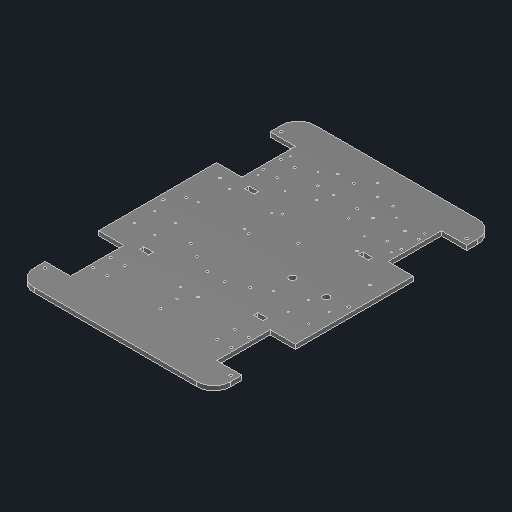
# Autodesk Inventor part: 부품7
Saved by Autodesk Inventor 2026.1 (Build 301233020, 233B)
## iProperties
Created: 2025-11-12
Part Number: 부품7
Material: ABS 플라스틱
Document SubType Name: Modeling
Designer: jaewook
Density: 1.06 g/cm^3
Appearance: 매끄러움 - 흰색
Author: jaewook
Autodesk Inventor part; units mm, degrees
ref_plane "YZ Plane" through (0, 0, 0) normal (1, 0, 0) x (0, 1, 0)
ref_plane "XZ Plane" through (0, 0, 0) normal (0, 1, 0) x (-1, 0, 0)
ref_plane "XY Plane" through (0, 0, 0) normal (0, 0, 1) x (1, 0, 0)
sketch "스케치1" plane through (0, 0, 0) normal (0, 1, 0) x (-1, 0, 0)
  line L0 (145, 250) -> (-145, 250)
  line L1 (-175, 220) -> (-175, -220)
  line L2 (-145, -250) -> (145, -250)
  line L3 (175, -220) -> (175, 220)
  line L4 (175, 250) -> (-175, -250) construction
  line L5 (-175, 250) -> (175, -250) construction
  arc A0 (145, -250) -> (175, -220) centre (145, -220) ccw
  arc A1 (-175, -220) -> (-145, -250) centre (-145, -220) ccw
  arc A2 (-145, 250) -> (-175, 220) centre (-145, 220) ccw
  arc A3 (175, 220) -> (145, 250) centre (145, 220) ccw
  line L6 (0, 0) -> (0, -150)
  line L7 (0, 0) -> (-113, 0)
  line L8 (175, -200) -> (130, -200)
  line L9 (130, -200) -> (130, -105)
  line L10 (130, -105) -> (175, -105)
  line L11 (175, -105) -> (175, -200)
  line L12 (-175, -200) -> (-130, -200)
  line L13 (-130, -200) -> (-130, -105)
  line L14 (-130, -105) -> (-175, -105)
  line L15 (-175, -105) -> (-175, -200)
  line L16 (175, 200) -> (130, 200)
  line L17 (130, 200) -> (130, 105)
  line L18 (130, 105) -> (175, 105)
  line L19 (175, 105) -> (175, 200)
  line L20 (-175, 200) -> (-130, 200)
  line L21 (-130, 105) -> (-175, 105)
  line L22 (-175, 105) -> (-175, 200)
  line L23 (-130, 200) -> (-130, 105)
  point P0 (-175, 200)
  point P1 (-175, 105)
  point P2 (-175, -105)
  point P3 (-175, -200)
  point P4 (175, 105)
  point P5 (175, 200)
  dimension "d0" = 350
  dimension "d1" = 500
  dimension "d2" = 30
  dimension "d4" = 95
  dimension "d5" = 45
  dimension "d6" = 50
  dimension "d9" = 50
  dimension "d10" = 45
  dimension "d11" = 95
  constraints: 48 end point, 12 symmetric about line, 9 point on line, 8 point on circle, 8 tangent, 4 centre point, 4 parallel, 3 equal radius, 3 horizontal, 2 midpoint, 2 perpendicular, 1 vertical
  measures "d0" distance of L5.end L4.end
  measures "d1" distance of L4.end L5.start
  measures "d2" radius of A0
  measures "d4" distance of L8.end L9.end
  measures "d5" distance of L9.end L10.end
  measures "d6" distance between parallel lines of L8 L2
  measures "d9" distance between parallel lines of L0 L16
  measures "d10" distance of L16.start L16.end
  measures "d11" distance of L16.end L17.end
extrude "돌출1" add sketch "스케치1" along normal blind 8 contours A3 L3 L16 L17 L18 L10 L9 L8 A0 L2 A1 L1 L12 L13 L14 L21 L23 L20 A2 L0
sketch "스케치3" plane through (0, 8, 0) normal (0, 1, 0) x (1, 0, 0)
  line L0 (175, -105) -> (175, 105) projected
  circle A0 centre (0, -85) radius 103.75 projected
  circle A1 centre (0, -85) radius 85
  line L1 (0, -85) -> (0, -170) construction
  circle A2 centre (0, -170) radius 2
  circle A3 centre (73.6122, -42.5) radius 2
  circle A4 centre (-73.6122, -42.5) radius 2
  point P0 (0, 0)
  dimension "d12" = 170
  dimension "d13" = 4
  dimension "d16" = 360
  constraints: 3 centre point, 2 coincident, 2 end point, 1 parallel, 1 vertical alignment, 9 other
  measures "d13" diameter of A2
extrude "돌출2" cut sketch "스케치3" against normal blind 10 contours A3 A1 | A1 A3 | A2 A1 | A1 A2 | A4 A1 | A1 A4
sketch "스케치4" plane through (0, 8, 0) normal (0, 1, 0) x (1, 0, 0)
  arc A0 (-175, -220) -> (-145, -250) centre (-145, -220) ccw projected
  line L0 (145, -250) -> (-145, -250) projected
  arc A1 (145, -250) -> (175, -220) centre (145, -220) ccw projected
  line L1 (175, 220) -> (175, -220) projected
  arc A2 (175, 220) -> (145, 250) centre (145, 220) ccw projected
  line L2 (-145, 250) -> (145, 250) projected
  arc A3 (-145, 250) -> (-175, 220) centre (-145, 220) ccw projected
  line L3 (-175, -220) -> (-175, 220) projected
  circle A4 centre (0, 175) radius 36 projected
  circle A5 centre (0, -85) radius 103.75 projected
  line L4 (-10, -75.2) -> (10, -75.2)
  line L5 (10, -75.2) -> (10, -115.2)
  line L6 (10, -115.2) -> (-10, -115.2)
  line L7 (-10, -115.2) -> (-10, -75.2)
  line L8 (0, -85) -> (0, -68) construction
  line L9 (-10, -95.2) -> (10, -95.2) construction
  line L10 (-10, -75.2) -> (-10, -67.7)
  line L11 (-10, -67.7) -> (10, -67.7)
  line L12 (10, -67.7) -> (10, -75.2)
  circle A6 centre (-5, -70.9) radius 2.5
  line L13 (-0.05, -69.45) -> (-0.05, -77.45)
  circle A7 centre (4.9, -70.9) radius 2.5
  line L14 (0, -105.4) -> (0, -122.4) construction
  line L15 (-10, -115.2) -> (-10, -122.7)
  line L16 (-10, -122.7) -> (10, -122.7)
  line L17 (10, -122.7) -> (10, -115.2)
  circle A8 centre (-5, -119.5) radius 2.5
  line L18 (-0.05, -120.95) -> (-0.05, -112.95)
  circle A9 centre (4.9, -119.5) radius 2.5
  point P0 (0, 0)
  dimension "d20" = 9.8
  dimension "d21" = 40
  dimension "d22" = 20
  dimension "d23" = 27.5
  dimension "d25" = 5
  dimension "d26" = 4.95
  dimension "d27" = 24.3
  dimension "d28" = 5
  constraints: 30 end point, 9 symmetric about line, 4 centre point, 3 perpendicular, 3 vertical, 2 midpoint, 2 parallel, 1 horizontal, 4 other
  measures "d20" distance from line of L8.start L4
  measures "d21" distance of L4.end L5.end
  measures "d22" distance of L4.start L4.end
  measures "d23" distance between parallel lines of L9 L11
  measures "d25" distance from line of A6.centre L10
  measures "d26" distance from line of L13 A6.centre
  measures "d27" distance from line of L9 A6.centre
  measures "d28" diameter of A6
extrude "돌출3" cut sketch "스케치4" against normal blind 10 contours A6 | A7 | A8 | A9
sketch "스케치6" plane through (0, 8, 0) normal (0, 1, 0) x (1, 0, 0)
  circle A0 centre (0, -170) radius 2 projected
  circle A1 centre (73.6122, -42.5) radius 2 projected
  circle A2 centre (-73.6122, -42.5) radius 2 projected
  line L0 (175, -105) -> (175, 105) projected
  line L1 (130, 105) -> (130, 200) projected
  line L2 (145, 250) -> (-145, 250) projected
  circle A3 centre (47.6412, -57.517) radius 2 projected
  circle A4 centre (-47.6216, -57.483) radius 2 projected
  circle A5 centre (-0.0196, -140) radius 2 projected
  circle A6 centre (0, 216.4634) radius 1.9 projected
  circle A7 centre (-28.4775, 136.4634) radius 1.9 projected
  circle A8 centre (28.4775, 136.4634) radius 1.9 projected
  circle A9 centre (123, 166.7672) radius 2.75 construction
  circle A10 centre (98, 166.7672) radius 2.75 construction
  circle A11 centre (98, 135.7672) radius 2.75 construction
  circle A12 centre (123, 135.7672) radius 2.75 construction
  circle A13 centre (123, 135.7672) radius 2
  circle A14 centre (123, 166.7672) radius 2
  circle A15 centre (98, 166.7672) radius 2
  circle A16 centre (98, 135.7672) radius 2
  line L3 (98, 135.7672) -> (98, 166.7672) construction
  line L4 (98, 166.7672) -> (123, 166.7672) construction
  line L5 (123, 166.7672) -> (123, 135.7672) construction
  line L6 (123, 151.2672) -> (98, 151.2672) construction
  circle A17 centre (119, 122.2672) radius 1.25
  circle A18 centre (70, 122.2672) radius 1.25
  line L7 (119, 122.2672) -> (70, 122.2672) construction
  line L8 (94.5, 122.2672) -> (94.5, 130) construction
  circle A19 centre (119, 180.2672) radius 1.25
  circle A20 centre (70, 180.2672) radius 1.25
  circle A21 centre (0.0018, 119.3) radius 3.75 projected
  circle A22 centre (0, 175) radius 33.15 projected
  line L9 (0.0018, 119.3) -> (0, 175) construction
  circle A23 centre (-118.9966, 122.2596) radius 1.25
  circle A24 centre (-69.9966, 122.2627) radius 1.25
  circle A25 centre (-70.0003, 180.2627) radius 1.25
  circle A26 centre (-119.0003, 180.2596) radius 1.25
  line L10 (175, -10) -> (155, -10) construction
  line L11 (155, -10) -> (155, 10) construction
  line L12 (155, 10) -> (175, 10) construction
  line L13 (175, 10) -> (175, -10) construction
  line L14 (0, 0) -> (-57, 0) construction
  line L15 (175, -10) -> (155, 10) construction
  line L16 (175, 10) -> (155, -10) construction
  circle A27 centre (165, 0) radius 2.5
  line L17 (0, 0) -> (0, -38) construction
  circle A28 centre (-165, 0) radius 2.5
  circle A29 centre (164.9933, 210) radius 2.5
  circle A30 centre (-165.0067, 210) radius 2.5
  circle A31 centre (165.0067, -210) radius 2.5
  circle A32 centre (-164.9933, -210) radius 2.5
  circle A33 centre (15.5, -71.3) radius 2 projected
  circle A34 centre (-15.5, -71.3) radius 2 projected
  circle A35 centre (15.5, -119.1) radius 2 projected
  circle A36 centre (-15.5, -119.1) radius 2 projected
  line L18 (123, 135.7672) -> (98, 135.7672) construction
  circle A37 centre (-122.9995, 166.7594) radius 2.75 construction
  circle A38 centre (-97.9995, 166.761) radius 2.75 construction
  circle A39 centre (-97.9975, 135.761) radius 2.75 construction
  circle A40 centre (-122.9975, 135.7594) radius 2.75 construction
  circle A41 centre (-122.9975, 135.7594) radius 2
  circle A42 centre (-122.9995, 166.7594) radius 2
  circle A43 centre (-97.9995, 166.761) radius 2
  circle A44 centre (-97.9975, 135.761) radius 2
  line L19 (-97.9975, 135.761) -> (-97.9995, 166.761) construction
  line L20 (-97.9995, 166.761) -> (-122.9995, 166.7594) construction
  line L21 (-122.9995, 166.7594) -> (-122.9975, 135.7594) construction
  line L22 (-122.9985, 151.2594) -> (-97.9985, 151.261) construction
  line L23 (-122.9975, 135.7594) -> (-97.9975, 135.761) construction
  circle A45 centre (123, -166.7672) radius 2.75 construction
  circle A46 centre (98, -166.7672) radius 2.75 construction
  circle A47 centre (98, -135.7672) radius 2.75 construction
  circle A48 centre (123, -135.7672) radius 2.75 construction
  circle A49 centre (123, -135.7672) radius 2
  circle A50 centre (123, -166.7672) radius 2
  circle A51 centre (98, -166.7672) radius 2
  circle A52 centre (98, -135.7672) radius 2
  line L24 (98, -135.7672) -> (98, -166.7672) construction
  line L25 (98, -166.7672) -> (123, -166.7672) construction
  line L26 (123, -166.7672) -> (123, -135.7672) construction
  line L27 (123, -151.2672) -> (98, -151.2672) construction
  line L28 (123, -135.7672) -> (98, -135.7672) construction
  circle A53 centre (-122.9975, -135.7594) radius 2.75 construction
  circle A54 centre (-122.9975, -135.7594) radius 2
  line L29 (-122.9975, -135.7594) -> (-97.9975, -135.761) construction
  circle A55 centre (-97.9975, -135.761) radius 2
  circle A56 centre (-97.9975, -135.761) radius 2.75 construction
  circle A57 centre (-122.9995, -166.7594) radius 2.75 construction
  line L30 (-122.9985, -151.2594) -> (-97.9985, -151.261) construction
  line L31 (-122.9995, -166.7594) -> (-122.9975, -135.7594) construction
  line L32 (-97.9975, -135.761) -> (-97.9995, -166.761) construction
  line L33 (-97.9995, -166.761) -> (-122.9995, -166.7594) construction
  circle A58 centre (-97.9995, -166.761) radius 2
  circle A59 centre (-97.9995, -166.761) radius 2.75 construction
  circle A60 centre (-122.9995, -166.7594) radius 2
  circle A61 centre (4.9, -70.9) radius 2.5 projected
  circle A62 centre (-5, -119.5) radius 2.5 projected
  circle A63 centre (-5, -70.9) radius 2.5 projected
  circle A64 centre (4.9, -119.5) radius 2.5 projected
  circle A65 centre (0, -170) radius 2 projected
  circle A66 centre (73.6122, -42.5) radius 2 projected
  circle A67 centre (-73.6122, -42.5) radius 2 projected
  line L34 (175, -220) -> (175, -200) projected
  line L35 (175, -200) -> (130, -200) projected
  line L36 (130, -200) -> (130, -105) projected
  line L37 (130, -105) -> (175, -105) projected
  line L38 (175, -105) -> (175, 105) projected
  line L39 (175, 105) -> (130, 105) projected
  line L40 (130, 105) -> (130, 200) projected
  line L41 (130, 200) -> (175, 200) projected
  line L42 (175, 200) -> (175, 220) projected
  arc A68 (175, 220) -> (145, 250) centre (145, 220) ccw projected
  line L43 (145, 250) -> (-145, 250) projected
  arc A69 (-145, 250) -> (-175, 220) centre (-145, 220) ccw projected
  line L44 (-175, 220) -> (-175, 200) projected
  line L45 (-175, 200) -> (-130, 200) projected
  line L46 (-130, 200) -> (-130, 105) projected
  line L47 (-130, 105) -> (-175, 105) projected
  line L48 (-175, 105) -> (-175, -105) projected
  line L49 (-175, -105) -> (-130, -105) projected
  line L50 (-130, -105) -> (-130, -200) projected
  line L51 (-130, -200) -> (-175, -200) projected
  line L52 (-175, -200) -> (-175, -220) projected
  arc A70 (-175, -220) -> (-145, -250) centre (-145, -220) ccw projected
  line L53 (-145, -250) -> (145, -250) projected
  arc A71 (145, -250) -> (175, -220) centre (145, -220) ccw projected
  circle A72 centre (28.4775, 136.4634) radius 1.5
  circle A73 centre (-28.4775, 136.4634) radius 1.5
  circle A74 centre (0, 216.4634) radius 1.5
  dimension "d39" = 4
  dimension "d41" = 4
  dimension "d42" = 4
  dimension "d47" = 2.5
  dimension "d49" = 4
  dimension "d51" = 49
  dimension "d52" = 2.5
  dimension "d57" = 20
  dimension "d58" = 20
  dimension "d59" = 5
  dimension "d62" = 330
  dimension "d65" = 210
  dimension "d69" = 7
  dimension "d70" = 114.2328
  dimension "d71" = 25
  dimension "d72" = 4
  dimension "d73" = 31
  dimension "d74" = 25
  dimension "d75" = 29
  dimension "d149" = 3
  dimension "d150" = 3
  dimension "d151" = 3
  constraints: 62 end point, 49 centre point, 39 symmetric about line, 24 coincident, 5 horizontal, 4 midpoint, 4 parallel, 1 horizontal alignment, 1 perpendicular, 1 point on line, 1 vertical, 1 vertical alignment, 42 other
  measures "d39" diameter of A13
  measures "d41" diameter of A14
  measures "d42" diameter of A15
  measures "d47" diameter of A17
  measures "d49" horizontal distance of L5.end L7.start
  measures "d51" distance of L7.start L7.end
  measures "d52" diameter of A18
  measures "d57" distance of L11.end L12.end
  measures "d58" distance of L10.end L11.end
  measures "d59" diameter of A27
  measures "d62" distance of A27.centre A28.centre
  measures "d65" distance of A27.centre A29.centre
  measures "d69" distance from line of L1 L5.end
  measures "d70" distance from line of L2 L5.end
  measures "d71" distance between centres of A13 A16
  measures "d72" diameter of A16
  measures "d73" distance of L4.end L5.end
  measures "d74" distance of L3.end L4.end
  measures "d75" distance from line of L6 L7.start
  measures "d149" diameter of A72
  measures "d150" diameter of A73
  measures "d151" diameter of A74
extrude "돌출4" cut sketch "스케치6" against normal blind 10 contours A0 | A1 | A2 | A3 | A4 | A5 | A13 | A14 | A15 | A16 | A17 | A18 | A19 | A20 | A23 | A24 | A25 | A26 | A27 | A28 | A29 | A30 | A31 | A32 | A33 | A34 | A35 | A36 | A41 | A42 | A43 | A44 | A49 | A50 | A51 | A52 | A54 | A55 | A58 | A60 | A72 | A73 | A74
sketch "스케치7" plane through (0, 8, 0) normal (0, 1, 0) x (1, 0, 0)
  circle A0 centre (4.9, -70.9) radius 2.5 projected
  circle A1 centre (-5, -119.5) radius 2.5 projected
  circle A2 centre (-5, -70.9) radius 2.5 projected
  circle A3 centre (4.9, -119.5) radius 2.5 projected
  point P0 (0, 0)
extrude "돌출5" add sketch "스케치7" against normal blind 8
sketch "스케치8" plane through (0, 8, 0) normal (0, 1, 0) x (1, 0, 0)
  circle A0 centre (123, -166.7672) radius 2 projected
  circle A1 centre (-122.9975, -135.7594) radius 2 projected
  circle A2 centre (-97.9975, 135.761) radius 2 projected
  circle A3 centre (-15.5, -71.3) radius 2 projected
  circle A4 centre (-165.0067, 210) radius 2.5 projected
  circle A5 centre (-119.0003, 180.2596) radius 1.25 projected
  circle A6 centre (119, 122.2672) radius 1.25 projected
  circle A7 centre (123, 135.7672) radius 2 projected
  circle A8 centre (-0.0196, -140) radius 2 projected
  circle A9 centre (123, 166.7672) radius 2 projected
  circle A10 centre (70, 122.2672) radius 1.25 projected
  circle A11 centre (-69.9966, 122.2627) radius 1.25 projected
  circle A12 centre (165, 0) radius 2.5 projected
  circle A13 centre (165.0067, -210) radius 2.5 projected
  circle A14 centre (15.5, -119.1) radius 2 projected
  circle A15 centre (-97.9995, 166.761) radius 2 projected
  circle A16 centre (-97.9995, -166.761) radius 2 projected
  circle A17 centre (98, -166.7672) radius 2 projected
  circle A18 centre (123, -135.7672) radius 2 projected
  circle A19 centre (-97.9975, -135.761) radius 2 projected
  circle A20 centre (-122.9975, 135.7594) radius 2 projected
  circle A21 centre (15.5, -71.3) radius 2 projected
  circle A22 centre (164.9933, 210) radius 2.5 projected
  circle A23 centre (-70.0003, 180.2627) radius 1.25 projected
  circle A24 centre (119, 180.2672) radius 1.25 projected
  circle A25 centre (98, 135.7672) radius 2 projected
  circle A26 centre (-47.6216, -57.483) radius 2 projected
  circle A27 centre (47.6412, -57.517) radius 2 projected
  circle A28 centre (98, 166.7672) radius 2 projected
  circle A29 centre (70, 180.2672) radius 1.25 projected
  circle A30 centre (-118.9966, 122.2596) radius 1.25 projected
  circle A31 centre (-165, 0) radius 2.5 projected
  circle A32 centre (-164.9933, -210) radius 2.5 projected
  circle A33 centre (-15.5, -119.1) radius 2 projected
  circle A34 centre (-122.9995, 166.7594) radius 2 projected
  circle A35 centre (-122.9995, -166.7594) radius 2 projected
  circle A36 centre (98, -135.7672) radius 2 projected
  circle A37 centre (0, -170) radius 2 projected
  circle A38 centre (73.6122, -42.5) radius 2 projected
  circle A39 centre (-73.6122, -42.5) radius 2 projected
  line L0 (175, -105) -> (175, 105) projected
  line L1 (130, 105) -> (130, 200) projected
  line L2 (145, 250) -> (-145, 250) projected
  line L3 (-130, 105) -> (-175, 105) projected
  circle A40 centre (150, 53) radius 2
  line L4 (21, 194.9548) -> (49.5, 194.9548) construction
  line L5 (49.5, 194.9548) -> (49.5, 158.9548) construction
  line L6 (49.5, 158.9548) -> (21, 158.9548) construction
  line L7 (21, 158.9548) -> (21, 194.9548) construction
  circle A41 centre (21, 194.9548) radius 2
  circle A42 centre (49.5, 194.9548) radius 2
  circle A43 centre (49.5, 158.9548) radius 2
  circle A44 centre (21, 158.9548) radius 2
  line L8 (150, 53) -> (22, 53) construction
  line L9 (86, 53) -> (86, 93.5) construction
  circle A45 centre (86, 93.5) radius 2
  circle A46 centre (22, 53) radius 2
  line L10 (0, 175) -> (0, 0) construction
  circle A47 centre (-21, 194.9548) radius 2
  circle A48 centre (-49.5, 194.9548) radius 2
  circle A49 centre (-49.5, 158.9548) radius 2
  circle A50 centre (-21, 158.9548) radius 2
  line L11 (155, -61.5) -> (118.5, -61.5) construction
  line L12 (118.5, -61.5) -> (118.5, -25) construction
  line L13 (118.5, -25) -> (155, -25) construction
  line L14 (155, -25) -> (155, -61.5) construction
  circle A51 centre (155, -25) radius 1.5
  circle A52 centre (118.5, -25) radius 1.5
  circle A53 centre (155, -61.5) radius 1.5
  circle A54 centre (118.5, -61.5) radius 1.5
  circle A55 centre (-155, -25) radius 1.5
  circle A56 centre (-118.5, -25) radius 1.5
  circle A57 centre (-155, -61.5) radius 1.5
  circle A58 centre (-118.5, -61.5) radius 1.5
  circle A59 centre (0, -85) radius 85 construction
  line L15 (-136.977, 80) -> (-32.377, 80) construction
  line L16 (-32.377, 80) -> (-32.377, 23.584) construction
  line L17 (-32.377, 23.584) -> (-136.977, 23.584) construction
  line L18 (-136.977, 23.584) -> (-136.977, 80) construction
  circle A60 centre (-123.133, 76) radius 1.5
  circle A61 centre (-48, 76) radius 1.5
  circle A62 centre (-47.999, 27.584) radius 1.5
  circle A63 centre (-130.626, 27.584) radius 1.5
  line L19 (93, 97.5) -> (110, 97.5)
  line L20 (110, 97.5) -> (110, 89.5)
  line L21 (110, 89.5) -> (93, 89.5)
  line L22 (93, 89.5) -> (93, 97.5)
  line L23 (105, 0) -> (0, 0) construction
  line L24 (-93, 97.5) -> (-110, 97.5)
  line L25 (-110, 97.5) -> (-110, 89.5)
  line L26 (-110, 89.5) -> (-93, 89.5)
  line L27 (-93, 89.5) -> (-93, 97.5)
  line L28 (93, -97.5) -> (110, -97.5)
  line L29 (110, -97.5) -> (110, -89.5)
  line L30 (110, -89.5) -> (93, -89.5)
  line L31 (93, -89.5) -> (93, -97.5)
  line L32 (-110, -97.5) -> (-110, -89.5)
  line L33 (-110, -89.5) -> (-93, -89.5)
  line L34 (-93, -89.5) -> (-93, -97.5)
  line L35 (-93, -97.5) -> (-110, -97.5)
  line L36 (-148, 84) -> (-37, 84) construction
  line L37 (-37, 84) -> (-37, 23.75) construction
  line L38 (-37, 23.75) -> (-148, 23.75) construction
  line L39 (-148, 23.75) -> (-148, 84) construction
  circle A64 centre (-37, 84) radius 2
  circle A65 centre (-37, 23.75) radius 2
  circle A66 centre (-148, 84) radius 2
  circle A67 centre (-148, 23.75) radius 2
  circle A68 centre (70, -5) radius 6
  circle A69 centre (130, -5) radius 6
  line L40 (-155, -10) -> (-175, -10)
  line L41 (-175, -10) -> (-175, 10)
  line L42 (-175, 10) -> (-155, 10)
  line L43 (-155, 10) -> (-155, -10)
  line L44 (-155, -10) -> (-175, 10) construction
  line L45 (-175, -10) -> (-155, 10) construction
  dimension "d80" = 4
  dimension "d81" = 25
  dimension "d83" = 28.5
  dimension "d84" = 36
  dimension "d85" = 4
  dimension "d86" = 4
  dimension "d87" = 4
  dimension "d88" = 4
  dimension "d89" = 128
  dimension "d90" = 40.5
  dimension "d91" = 4
  dimension "d92" = 4
  dimension "d93" = 53
  dimension "d94" = 21
  dimension "d96" = 36.5
  dimension "d97" = 36.5
  dimension "d98" = 3
  dimension "d99" = 3
  dimension "d100" = 3
  dimension "d101" = 3
  dimension "d102" = 25
  dimension "d103" = 104.6
  dimension "d104" = 56.416
  dimension "d105" = 3
  dimension "d106" = 3
  dimension "d107" = 4
  dimension "d108" = 13.844
  dimension "d109" = 75.133
  dimension "d110" = 3
  dimension "d111" = 3
  dimension "d112" = 4
  dimension "d113" = 15.622
  dimension "d114" = 6.351
  dimension "d117" = 17
  dimension "d118" = 8
  dimension "d119" = 19.9548
  dimension "d120" = 75
  dimension "d121" = 20
  dimension "d122" = 7.5
  dimension "d123" = 111
  dimension "d124" = 60.25
  dimension "d125" = 4
  dimension "d126" = 4
  dimension "d127" = 4
  dimension "d128" = 4
  dimension "d129" = 37
  dimension "d130" = 48
  dimension "d131" = 21
  dimension "d132" = 29
  dimension "d136" = 53
  dimension "d137" = 70
  dimension "d140" = 12
  dimension "d141" = 12
  dimension "d142" = 60
  dimension "d144" = 45
  dimension "d145" = 20
  dimension "d146" = 20
  dimension "d147" = 20
  dimension "d148" = 20
  constraints: 84 end point, 30 centre point, 20 symmetric about line, 15 coincident, 12 parallel, 8 horizontal, 6 perpendicular, 3 horizontal alignment, 3 midpoint, 3 point on circle, 2 vertical, 1 tangent, 8 other
  measures "d80" diameter of A40
  measures "d81" distance from line of L0 A40.centre
  measures "d83" distance of L5.end L6.end
  measures "d84" distance of L4.end L5.end
  measures "d85" diameter of A41
  measures "d86" diameter of A42
  measures "d87" diameter of A43
  measures "d88" diameter of A44
  measures "d89" distance of L8.start L8.end
  measures "d90" distance of L9.start L9.end
  measures "d91" diameter of A45
  measures "d92" diameter of A46
  measures "d93" vertical distance of A12.centre A40.centre
  measures "d94" distance from line of L10 L4.start
  measures "d96" distance of L12.end L13.end
  measures "d97" distance of L11.end L12.end
  measures "d98" diameter of A51
  measures "d99" diameter of A52
  measures "d100" diameter of A53
  measures "d101" diameter of A54
  measures "d102" vertical distance of L13.end A12.centre
  measures "d103" distance of L16.end L17.end
  measures "d104" distance of L15.end L16.end
  measures "d105" diameter of A60
  measures "d106" diameter of A61
  measures "d107" distance from line of A60.centre L15
  measures "d108" distance from line of A60.centre L18
  measures "d109" distance of A61.centre A60.centre
  measures "d110" diameter of A62
  measures "d111" diameter of A63
  measures "d112" distance from line of L17 A62.centre
  measures "d113" distance from line of L16 A62.centre
  measures "d114" distance from line of L18 A63.centre
  measures "d117" distance of L20.end L21.end
  measures "d118" distance of L19.end L20.end
  measures "d119" vertical distance of L10.start L4.start
  measures "d120" distance from line of L2 L10.start
  measures "d121" distance from line of L1 L19.end
  measures "d122" vertical distance of L1.start L19.end
  measures "d123" distance of L37.end L38.end
  measures "d124" distance of L36.end L37.end
  measures "d125" diameter of A64
  measures "d126" diameter of A65
  measures "d127" diameter of A66
  measures "d128" diameter of A67
  measures "d129" distance from line of L10 A64.centre
  measures "d130" distance from line of L10 A61.centre
  measures "d131" distance from line of L3 L36.end
  measures "d132" distance from line of L3 A61.centre
  measures "d136" distance from line of L23.start L8
  measures "d137" distance from line of L0 L23.start
  measures "d140" diameter of A68
  measures "d141" diameter of A69
  measures "d142" distance of A69.centre A68.centre
  measures "d144" distance from line of L0 A69.centre
  measures "d145" distance from line of L0 L13.end
  measures "d146" distance of L41.end L42.end
  measures "d147" distance of L40.end L41.end
  measures "d148" distance from line of A69.centre L13
extrude "돌출6" cut sketch "스케치8" along normal through all both and the other way through all contours A0 | A1 | A2 | A3 | A4 | A5 | A6 | A7 | A8 | A9 | A10 | A11 | A12 | A13 | A14 | A15 | A16 | A17 | A18 | A19 | A20 | A21 | A22 | A23 | A24 | A25 | A26 | A27 | A28 | A29 | A30 | A31 | A32 | A33 | A34 | A35 | A36 | A37 | A38 | A39 | A40 | A41 | A42 | A43 | A44 | A45 | A46 | A47 | A48 | A49 | A50 | A51 | A52 | A53 | A54 | A55 | A56 | A57 | A58 | A60 | A61 | A62 | A63 | L19 L20 L21 L22 | L27 L26 L25 L24 | L31 L30 L29 L28 | L32 L33 L34 L35 | A64 | A65 | A66 | A67 | A68 | A69
equation "\"d39\" = d35"
equation "\"d41\" = d39"
equation "\"d42\" = d40"
equation "\"d52\" = d47"
equation "\"d35\" = d31"
equation "\"d40\" = d39"
equation "\"d31\" = 4"
